Autodesk Fusion 360 part; units mm, degrees
(part 3 of 3)
sketch "Sketch10" plane through (0, 0, 41.1) normal (0, 0, 1) x (-1, 0, 0)
  line L0 (-1.5, 10.3) -> (-1.5, 17.5)
  line L1 (-1.5, 17.5) -> (-8.5, 17.5)
  line L2 (-8.5, 17.5) -> (-8.5, 10.3)
  line L3 (-8.5, 10.3) -> (-1.5, 10.3)
  line L4 (-8.5, 10.3) -> (-1.5, 17.5)
  line L5 (-1.5, 10.3) -> (-8.5, 17.5)
  circle A0 centre (-5, 13.9) radius 1.65
  dimension "d107" = 3.3
  constraint coincident L2.end L3.start
  constraint coincident L0.end L1.start
  constraint coincident L0.start L3.end
  constraint coincident L1.end L2.start
  constraint midpoint L5 A0.centre
  measures "d107" diameter of A0
extrude "Extrude14" add sketch "Sketch10" along normal blind 4.3 contours L4 L5 A0 | L4 L5 A0 | L4 L5 A0 | L4 L5 A0
sketch "Sketch11" plane through (0, -18.85, 0) normal (0, -1, 0) x (1, 0, 0)
  line L0 (0, 42) -> (0, 6.5)
  line L1 (0, 6.5) -> (1.5, 6.5)
  line L2 (1.5, 6.5) -> (1.5, 27)
  line L3 (1.5, 27) -> (4.5, 27)
  line L4 (4.5, 27) -> (4.5, 34.3)
  line L5 (4.5, 34.3) -> (1.5, 34.3)
  line L6 (1.5, 34.3) -> (1.5, 42)
  line L7 (1.5, 42) -> (0, 42)
  line L8 (1.5, 34.3) -> (1.5, 27)
  line L9 (2, 32.5) -> (2, 29)
  arc A0 (2, 29) -> (4, 29) centre (3, 29) ccw
  line L10 (4, 29) -> (4, 32.5)
  arc A1 (4, 32.5) -> (2, 32.5) centre (3, 32.5) ccw
  line L11 (3, 32.5) -> (3, 29) construction
  line L12 (1.5, 34.3) -> (4.5, 34.3)
  line L13 (4.5, 27) -> (4.5, 34.3)
  line L14 (4.5, 27) -> (1.5, 27)
  dimension "d110" = 2
  constraint coincident L5.end L6.start
  constraint coincident L2.end L3.start
  constraint tangent L9 A0
  constraint tangent A0 L10
  constraint parallel L9 L10
  constraint tangent L10 A1
  constraint tangent L9 A1
  constraint vertical L11
  constraint coincident L4.end L5.start
  constraint coincident L3.end L4.start
  measures "d110" diameter of A0
extrude "Extrude15" cut sketch "Sketch11" against normal blind 5 contours L9 A0 L10 A1
sketch "Sketch12" plane through (0, -13.85, 0) normal (0, -1, 0) x (1, 0, 0)
  arc A0 (4, 32.5) -> (2, 32.5) centre (3, 32.5) ccw
  line L0 (2, 32.5) -> (2, 29)
  arc A1 (2, 29) -> (4, 29) centre (3, 29) ccw
  line L1 (4, 29) -> (4, 32.5)
  line L2 (2.5, 33) -> (2.8, 33)
  line L3 (2.8, 33) -> (2.8, 28.5)
  line L4 (2.8, 28.5) -> (2.5, 28.5)
  line L5 (2.5, 28.5) -> (2.5, 33)
  constraint horizontal L2
  constraint vertical L3
  constraint horizontal L4
  constraint vertical L5
extrude "Extrude16" add sketch "Sketch12" along normal blind 4.5 contours L2 L3 L4 L5
fillet "Fillet2" radius 2 2 edges at (4.5, -16.2, 27) (4.5, -16.2, 34.3)
extrude "Extrude17" cut sketch "Sketch7" against normal blind 32 contours A0 | A1 | A2
equation "d16 = d15"
equation "d18 = d17"
